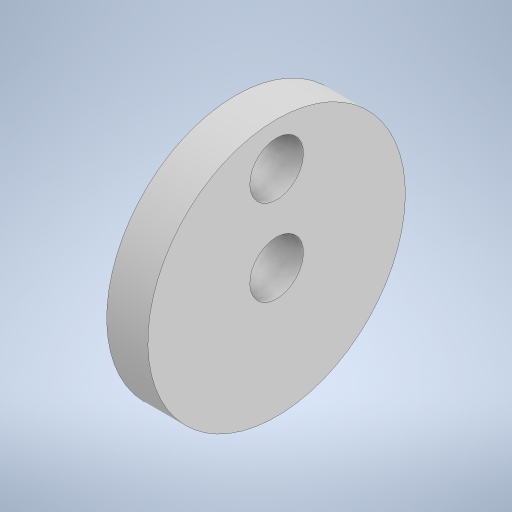
# Autodesk Inventor part: Crankshaft Crank Wheel
Saved by Autodesk Inventor 2023 (Build 270158000, 158)
## iProperties
Created: 2023-02-24
Part Number: Crankshaft Crank Wheel
Material: Generic
Document SubType Name: Modeling
Designer: tommy
Density: 1 g/cm^3
Appearance: Default
Author: tommy
Autodesk Inventor part; units mm, degrees
ref_plane "YZ Plane" through (0, 0, 0) normal (1, 0, 0) x (0, 1, 0)
ref_plane "XZ Plane" through (0, 0, 0) normal (0, 1, 0) x (-1, 0, 0)
ref_plane "XY Plane" through (0, 0, 0) normal (0, 0, 1) x (1, 0, 0)
sketch "Sketch1" plane through (0, 0, 0) normal (1, 0, 0) x (0, 1, 0)
  circle A0 centre (0, 0) radius 4.7625
  circle A1 centre (3.175, 0) radius 0.9922
  circle A2 centre (0, 0) radius 0.9922
  line L0 (0, 0) -> (3.175, 0)
  dimension "d0" = 9.525
  dimension "d1" = 1.9844
  dimension "d2" = 3.175
  dimension "d3" = 1.9844
  constraints: 3 centre point, 2 coincident, 2 end point, 1 horizontal
  measures "d0" diameter of A0
  measures "d1" diameter of A1
  measures "d2" distance of point (0, 0) L0.end
  measures "d3" diameter of A2
extrude "Extrusion1" add sketch "Sketch1" along normal blind 1.524
body "Solid1"
